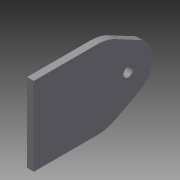
# Autodesk Inventor part: Suporte Motor
Saved by Autodesk Inventor 2015 (Build 190159000, 159)
## iProperties
Created: 2016-06-05
Part Number: Suporte Motor
Material: Generic
Document SubType Name: Modeling
Designer: EriveltonDell
Density: 1 g/cm^3
Appearance: Default
Author: EriveltonDell
Autodesk Inventor part; units mm, degrees
ref_plane "YZ Plane" through (0, 0, 0) normal (1, 0, 0) x (0, 1, 0)
ref_plane "XZ Plane" through (0, 0, 0) normal (0, 1, 0) x (-1, 0, 0)
ref_plane "XY Plane" through (0, 0, 0) normal (0, 0, 1) x (1, 0, 0)
sketch "Sketch3" plane through (0, 0, 0) normal (1, 0, 0) x (0, 1, 0)
  line L0 (0, 0) -> (56.36, 0)
  line L1 (56.36, 70) -> (0, 70)
  line L2 (0, 70) -> (0, 0)
  circle A0 centre (84, 35) radius 4.25
  line L3 (84, 35) -> (56.36, 35)
  line L4 (96, 53.4391) -> (74.4743, 64.9114)
  line L5 (94.3473, 15.5852) -> (72.8216, 4.1129)
  arc A1 (94.3473, 15.5852) -> (92.6159, 55.2427) centre (84, 35) ccw
  arc A2 (74.9172, 64.6754) -> (56.36, 70) centre (56.36, 35) ccw
  arc A3 (56.36, 0) -> (72.8216, 4.1129) centre (56.36, 35) ccw
  line L6 (84, 35) -> (71.3, 35)
  dimension "d31" = 8.5
  dimension "d33" = 27.64
  dimension "d35" = 12.7
  dimension "d41" = 84
  constraints: 14 end point, 6 point on circle, 4 centre point, 3 point on line, 2 coincident, 2 horizontal, 1 parallel, 1 tangent
  measures "d31" diameter of A0
  measures "d33" distance of L3.start L3.end
  measures "d35" distance of L3.start L6.end
  measures "d41" distance from line of L2 A0.centre
extrude "Extrusion3" add sketch "Sketch3" along normal blind 6
body "Solid2"
